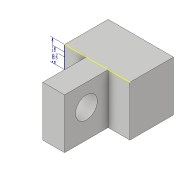
# Autodesk Inventor part: pusher
Saved by Autodesk Inventor 2019 (Build 230136000, 136)
## iProperties
Created: 2019-10-16
Part Number: pusher
Material: Generic
Document SubType Name: Sheet Metal
Designer: Admin
Density: 1 g/cm^3
Sheet Metal Rule: Default_mm
Appearance: Default
Author: Admin
Autodesk Inventor part; units mm, degrees
ref_plane "YZ Plane" through (0, 0, 0) normal (1, 0, 0) x (0, 1, 0)
ref_plane "XZ Plane" through (0, 0, 0) normal (0, 1, 0) x (-1, 0, 0)
ref_plane "XY Plane" through (0, 0, 0) normal (0, 0, 1) x (1, 0, 0)
sketch "Sketch1" plane through (0, 0, 0) normal (0, 0, 1) x (1, 0, 0)
  line L0 (0, 0) -> (30, 0)
  line L1 (30, 0) -> (30, 23)
  line L2 (30, 23) -> (0, 23)
  line L3 (0, 23) -> (0, 0)
  dimension "d0" = 30
  dimension "d1" = 23
  constraints: 8 end point, 2 parallel, 1 horizontal, 1 perpendicular
  measures "d0" distance of L2.end L1.end
  measures "d1" distance of L1.end L0.end
extrude "Extrusion1" add sketch "Sketch1" along normal blind 20
sketch "Sketch2" plane through (0, 0, 20) normal (0, 0, 1) x (1, 0, 0)
  line L0 (30, 23) -> (0, 23) projected
  line L1 (0, 23) -> (0, 13)
  line L2 (0, 23) -> (0, 0) projected
  dimension "d4" = 10
  constraints: 2 end point, 1 point on line
  measures "d4" distance of L0.end L1.end
sketch "Sketch3" plane through (0, 0, 20) normal (0, 0, 1) x (1, 0, 0)
  point P0 (0, 0)
sketch "Sketch4" plane through (0, 0, 20) normal (0, 0, 1) x (1, 0, 0)
  line L0 (0, 23) -> (0, 0) projected
  line L1 (0, 13) -> (0, 20)
  dimension "d5" = 7
  constraints: 2 end point, 2 point on line
  measures "d5" distance of L1.start L1.end
sketch "Sketch5" plane through (0, 0, 20) normal (0, 0, 1) x (1, 0, 0)
  line L0 (0, 23) -> (0, 0) projected
  line L1 (0, 13) -> (0, 18)
  dimension "d6" = 5
  constraints: 2 end point, 2 point on line
  measures "d6" distance of L1.start L1.end
sketch "Sketch6" plane through (0, 0, 20) normal (0, 0, 1) x (1, 0, 0)
  line L0 (0, 23) -> (10, 23)
  line L1 (30, 23) -> (0, 23) projected
  line L2 (10, 23) -> (20, 23)
  line L3 (0, 0) -> (30, 0) projected
  line L4 (10, 23) -> (20, 23)
  line L5 (20, 23) -> (20, 0)
  line L6 (20, 0) -> (10, 0)
  line L7 (10, 0) -> (10, 23)
  dimension "d7" = 10
  dimension "d8" = 10
  constraints: 12 end point, 3 point on line, 2 parallel, 1 horizontal, 1 perpendicular
  measures "d7" distance of L0.start L0.end
  measures "d8" distance of L0.end L2.end
extrude "Extrusion2" add sketch "Sketch6" along normal blind 20
sketch "Sketch7" plane through (20, 0, 20) normal (1, 0, 0) x (0, 0, -1)
  line L0 (0, 23) -> (-20, 23) projected
  line L1 (-20, 23) -> (-20, 13)
  line L2 (-20, 23) -> (-20, 0) projected
  line L3 (-20, 13) -> (-10, 13)
  circle A0 centre (-10, 13) radius 5
  point P0 (20, 0)
  dimension "d11" = 10
  dimension "d12" = 10
  dimension "d13" = 10
  constraints: 4 end point, 1 centre point, 1 coincident, 1 perpendicular, 1 point on line
  measures "d11" distance of L0.end L1.end
  measures "d12" distance of L1.end L3.end
  measures "d13" diameter of A0
extrude "Extrusion3" cut sketch "Sketch7" against normal blind 20
equation "\"BendRadius\" = Thickness"
equation "\"BendReliefWidth\" = Thickness"
equation "\"BendReliefDepth\" = 0.5 * Thickness"
equation "\"CornerReliefSize\" = 4 * Thickness"
equation "\"MinimumRemnant\" = 2 * Thickness"
equation "\"TransitionRadius\" = BendRadius"
equation "\"JacobiRadiusSize\" = BendRadius"
equation "\"GapSize\" = Thickness"
equation "\"Thickness\" = 0.5"
body "Solid1"
